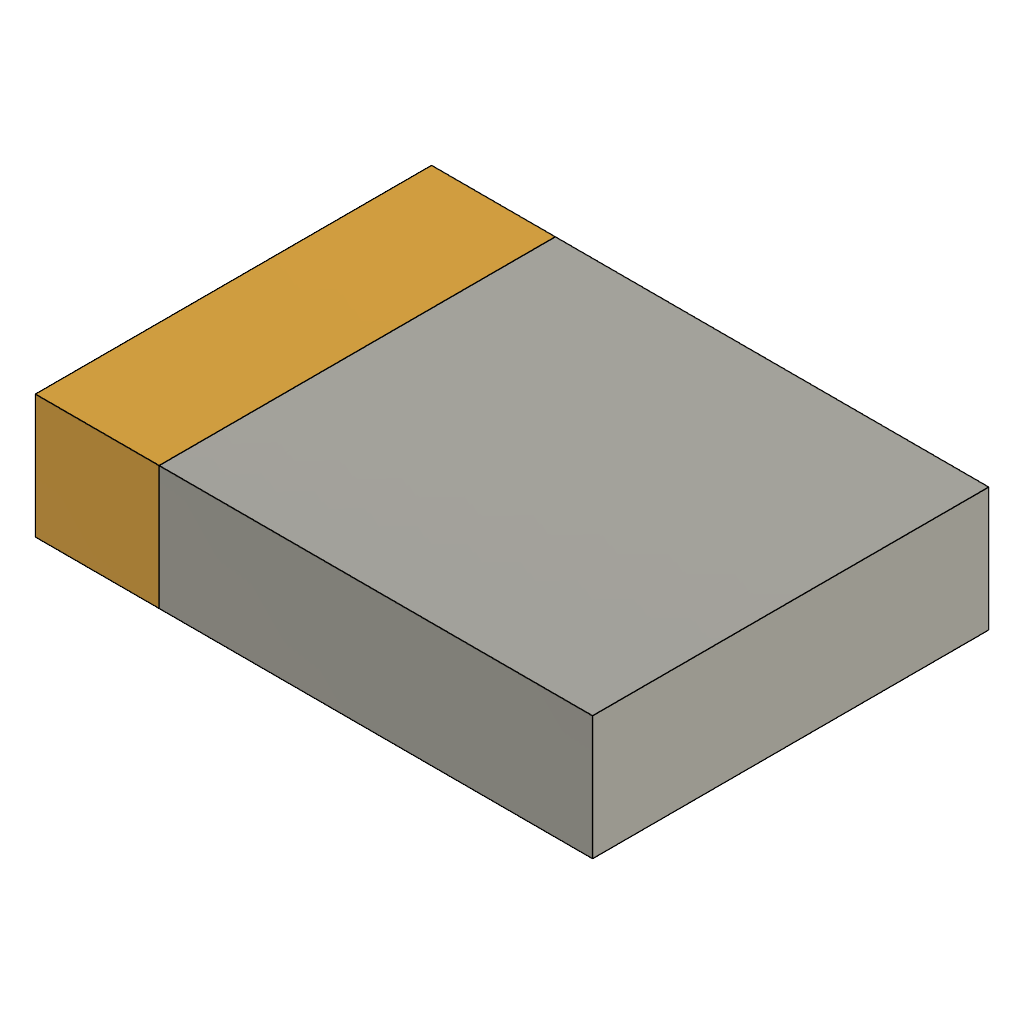
Device Body (Autodesk Fusion 360 archive; units mm, degrees)
design "1200 mAh Battery"
Autodesk Fusion 360 part; units mm, degrees
sketch "Sketch1" plane through (0, 0, 0) normal (0, 0, 1) x (1, 0, 0)
  line L0 (-22.5, 16) -> (22.5, 16)
  line L1 (22.5, 16) -> (22.5, -16)
  line L2 (22.5, -16) -> (-22.5, -16)
  line L3 (-22.5, -16) -> (-22.5, 16)
  line L4 (-22.5, 16) -> (22.5, -16) construction
  line L5 (22.5, 16) -> (-22.5, -16) construction
  dimension "d1" = 45
  dimension "d2" = 32
  constraint horizontal L0
  constraint perpendicular L0 L1
  constraint parallel L0 L2
  constraint parallel L1 L3
  constraint coincident L4 origin
  constraint coincident L5 origin
  measures "d1" distance of L1.end L2.end
  measures "d2" distance of L0.end L1.end
extrude "Extrude1" add sketch "Sketch1" along normal blind 10 makes body 1
ref_plane "WorkPlane1" through (-12.5, 0, 5) normal (-1, 0, 0) x (0, -1, 0)
split "Split1" by plane through (-12.5, 0, 5) normal (-1, 0, 0) bodies 1 makes body 2 at (-19.1667, 5.3333, 0)
